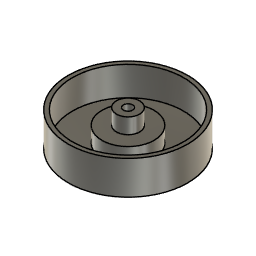
Wheel (Autodesk Fusion 360 design; units mm, degrees)
Autodesk Fusion 360 part; units mm, degrees
sketch "Sketch1" plane through (0, 0, 0) normal (0, 0, 1) x (1, 0, 0)
  circle A0 centre (0, 0) radius 15.45
  circle A1 centre (0, 0) radius 14.4
  circle A2 centre (0, 0) radius 6.75
  circle A3 centre (0, 0) radius 3
  circle A4 centre (0, 0) radius 1.2
  dimension "d24" = 30.9
  dimension "d25" = 28.8
  dimension "d26" = 13.5
  dimension "d27" = 6
  dimension "d28" = 2.4
  constraint coincident A0.centre A1.centre
  constraint concentric A0 A3
  constraint concentric A1 A4
  measures "d24" diameter of A0
  measures "d25" diameter of A1
  measures "d26" diameter of A2
  measures "d27" diameter of A3
  measures "d28" diameter of A4
extrude "Extrude1" add sketch "Sketch1" along normal blind 1.2 contours A1 makes body 1
extrude "Extrude2" add sketch "Sketch1" along normal blind 8.7 contours A0 bodies 1
extrude "Extrude3" add sketch "Sketch1" along normal blind 9.2 separate body contours A3 makes body 2
extrude "Extrude4" add sketch "Sketch1" along normal blind 5.2 contours A2 bodies 1 2
equation "d25 = 30.9 mm - 2.1 mm"
equation "d35 = 9.2 mm - 4 mm"
